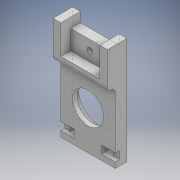
# Autodesk Inventor part: PISTON_bearing
Saved by Autodesk Inventor 2018 (Build 220112000, 112)
## iProperties
Created: 2026-07-08
Part Number: PISTON_bearing
Material: Generic
Document SubType Name: Modeling
Designer: neo
Density: 1 g/cm^3
Appearance: Default
Author: neo
Autodesk Inventor part; units mm, degrees
ref_plane "YZ Plane" through (0, 0, 0) normal (1, 0, 0) x (0, 1, 0)
ref_plane "XZ Plane" through (0, 0, 0) normal (0, 1, 0) x (-1, 0, 0)
ref_plane "XY Plane" through (0, 0, 0) normal (0, 0, 1) x (1, 0, 0)
sketch "Sketch1" plane through (0, 0, 0) normal (0, 1, 0) x (-1, 0, 0)
  line L0 (-1.5171, 15.4904) -> (-1.5171, -24.1277) construction
  line L1 (12.4829, 23.2632) -> (-15.5171, 23.2632)
  line L2 (-15.5171, 23.2632) -> (-15.5171, -31.7368)
  line L3 (-15.5171, -31.7368) -> (12.4829, -31.7368)
  line L4 (12.4829, -31.7368) -> (12.4829, 23.2632)
  line L5 (1.173, -11.7368) -> (-5.6801, -11.7368) construction
  circle A0 centre (-1.5171, -11.7368) radius 11
  line L6 (8.4829, 8.2632) -> (-11.5171, 8.2632)
  line L7 (-11.5171, 8.2632) -> (-11.5171, 23.2632)
  line L8 (-11.5171, 23.2632) -> (8.4829, 23.2632)
  line L9 (8.4829, 23.2632) -> (8.4829, 8.2632)
  point P0 (0, 0)
  dimension "d0" = 22
  dimension "d1" = 28
  dimension "d2" = 20
  dimension "d3" = 15
  dimension "d4" = 20
  dimension "d16" = 55
  constraints: 20 end point, 4 parallel, 3 horizontal, 3 point on line, 2 perpendicular, 1 centre point, 1 vertical, 2 other
  measures "d0" diameter of A0
  measures "d1" distance of L2.end L3.end
  measures "d2" distance of L6.start L6.end
  measures "d3" distance of L8.end L6.start
  measures "d4" distance between parallel lines of L3 L5
  measures "d16" distance of L1.end L2.end
extrude "Extrusion1" add sketch "Sketch1" along normal blind 10 contours L4 L3 L2 L1 L7 L6 L9
extrude "Extrusion2" add sketch "Sketch1" along normal blind 6.4 contours A0
sketch "Sketch2" plane through (0, 10, 0) normal (0, 1, 0) x (1, 0, 0)
  line L0 (11.5171, -8.2632) -> (-8.4829, -8.2632) projected
  line L1 (-8.4829, -8.2632) -> (11.5171, -8.2632)
  line L2 (11.5171, -8.2632) -> (11.5171, -18.2632)
  line L3 (11.5171, -18.2632) -> (-8.4829, -18.2632)
  line L4 (-8.4829, -18.2632) -> (-8.4829, -8.2632)
  point P0 (0, 0)
  dimension "d9" = 10
  constraints: 8 end point, 2 parallel, 1 horizontal, 1 perpendicular
  measures "d9" distance of L3.end L0.end
extrude "Extrusion3" add sketch "Sketch2" against normal blind 5
sketch "Sketch3" plane through (15.5171, 0, 23.2632) normal (1, 0, 0) x (0, 0, -1)
  line L0 (0, 0) -> (55, 0) construction
  line L1 (55, 0) -> (55, 10) construction
  line L2 (0, 10) -> (55, 10) construction
  line L3 (0, 0) -> (0, 10) construction
  line L4 (55, 0) -> (19, 0)
  line L5 (19, 0) -> (19, 4)
  line L6 (19, 4) -> (55, 4)
  line L7 (55, 4) -> (55, 0)
  line L8 (24, 6.4) -> (46, 6.4) construction
  line L9 (24, 10) -> (46, 10) construction
  point P0 (23.2632, 0)
  dimension "d12" = 6
  dimension "d17" = 5
  constraints: 8 end point, 2 parallel, 1 horizontal, 1 perpendicular
  measures "d12" distance between parallel lines of L2 L6
  measures "d17" distance from line of L8.start L5
extrude "Extrusion4" cut sketch "Sketch3" against normal through all
sketch "Sketch4" plane through (15.5171, 4, -31.7368) normal (0, -1, 0) x (1, 0, 0)
  line L0 (1.7907, 5) -> (-31.4365, 5) construction
  line L1 (0, 0) -> (-28, 0) construction
  line L2 (-3, 7) -> (-7, 7)
  line L3 (-7, 7) -> (-7, 3)
  line L4 (-7, 3) -> (-3, 3)
  line L5 (-3, 3) -> (-3, 7)
  line L6 (-5, 9.5929) -> (-5, 0.7775) construction
  line L7 (0, 36) -> (0, 0) construction
  line L8 (-14, 47.2272) -> (-14, 7.6092) construction
  line L9 (-25, 7) -> (-21, 7)
  line L10 (-21, 7) -> (-21, 3)
  line L11 (-21, 3) -> (-25, 3)
  line L12 (-25, 3) -> (-25, 7)
  point P0 (-15.5171, 31.7368)
  dimension "d18" = 5
  dimension "d19" = 4
  dimension "d20" = 5
  constraints: 20 end point, 4 symmetric about line, 2 horizontal, 2 parallel, 2 perpendicular, 1 vertical, 2 other
  measures "d18" distance between parallel lines of L1 L0
  measures "d19" distance of L3.end L4.end
  measures "d20" distance between parallel lines of L7 L6
extrude "Extrusion5" cut sketch "Sketch4" against normal through all
fillet "Fillet1" radius 2 2 edges at (1.5171, 4, 4.2632) (1.5171, 0, 4.2632)
sketch "Sketch5" plane through (0, 10, 0) normal (0, 1, 0) x (1, 0, 0)
  line L0 (11.5171, -18.2632) -> (-8.4829, -18.2632) construction
  line L1 (1.5171, -18.2632) -> (1.5171, -0.9417) construction
  circle A0 centre (1.5171, -13.2632) radius 1.5
  point P0 (0, 0)
  dimension "d24" = 3
  dimension "d25" = 5
  constraints: 2 end point, 1 centre point, 1 midpoint, 1 point on line, 1 vertical
  measures "d24" diameter of A0
  measures "d25" distance from line of L0 A0.centre
extrude "Extrusion6" cut sketch "Sketch5" against normal through all
sketch "Sketch6" plane through (1.5171, 6.4, -11.7368) normal (0, 1, 0) x (1, 0, 0)
  circle A0 centre (0, 0) radius 11 construction
  circle A1 centre (0, 0) radius 8
  point P0 (-1.5171, -11.7368)
  dimension "d28" = 3
  constraints: 1 centre point, 1 coincident
  measures "d28" radial gap between concentric circles of A0 A1
extrude "Extrusion7" cut sketch "Sketch6" against normal through all
sketch "Sketch8" plane through (-12.4829, 4, -31.7368) normal (0, -1, 0) x (1, 0, 0)
  circle A0 centre (14, 20) radius 8 construction
  line L0 (0, 34) -> (28, 34) construction
  line L1 (0, 0) -> (0, 34) construction
  line L2 (28, 0) -> (0, 0) construction
  line L3 (28, 34) -> (28, 0) construction
  line L4 (21, 3) -> (21, 7) construction
  line L5 (21, 7) -> (25, 7) construction
  line L6 (25, 7) -> (25, 3) construction
  line L7 (25, 3) -> (21, 3) construction
  line L8 (3, 3) -> (3, 7) construction
  line L9 (3, 7) -> (7, 7) construction
  line L10 (7, 7) -> (7, 3) construction
  line L11 (7, 3) -> (3, 3) construction
  line L12 (3, 7) -> (-3.7941, 7)
  line L13 (-3.7941, 7) -> (-3.7941, 3)
  line L14 (-3.7941, 3) -> (3, 3)
  line L15 (3, 3) -> (3, 7)
  line L16 (25, 7) -> (32.0495, 7)
  line L17 (32.0495, 7) -> (32.0495, 3)
  line L18 (32.0495, 3) -> (25, 3)
  line L19 (25, 3) -> (25, 7)
  point P0 (12.4829, 31.7368)
  constraints: 16 end point, 4 parallel, 2 horizontal, 2 perpendicular
extrude "Extrusion9" cut sketch "Sketch8" against normal blind 2
body "Solid1"
